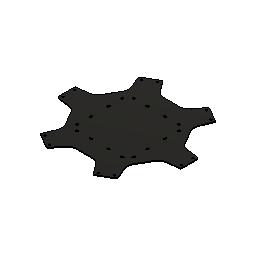
F550 Bottom Plate v5 (Autodesk Fusion 360 design; units mm, degrees)
Autodesk Fusion 360 part; units mm, degrees
sketch "Sketch1" plane through (0, 0, 0) normal (0, 0, 1) x (1, 0, 0)
  circle A0 centre (0, 0) radius 275 construction
  line L0 (-110, -15.85) -> (-110, 15.85)
  circle A1 centre (-105, 10.5) radius 1.75
  circle A2 centre (-105, -10.5) radius 1.75
  line L1 (-105, 10.5) -> (-105, -10.5) construction
  line L2 (0, 0) -> (-67.55, 39)
  line L3 (0, 0) -> (-67.55, -39)
  line L4 (0, 0) -> (-105, 0) construction
  line L5 (-110, -15.85) -> (-87.3994, -18.594)
  line L6 (-67.55, -39) -> (-74.3532, -27.2164)
  arc A3 (-74.3532, -27.2164) -> (-87.3994, -18.594) centre (-89.5087, -35.9664) ccw
  line L7 (-110, 15.85) -> (-87.3994, 18.594)
  arc A4 (-87.3994, 18.594) -> (-74.3532, 27.2164) centre (-89.5087, 35.9664) ccw
  line L8 (-67.55, 39) -> (-74.3532, 27.2164)
  point P0 (-110, 0)
  point P1 (-105, 0)
  point P2 (-275, 0)
  point P3 (-107, -10)
  point P4 (-107, 10)
  point P5 (-107, 0)
  dimension "d1" = 550
  dimension "d2" = 21
  dimension "d3" = 5
  dimension "d5" = 170
  dimension "d6" = 3.5
  dimension "d7" = 31.7
  dimension "d8" = 30
  dimension "d9" = 30
  dimension "d10" = 78
  dimension "d13" = 20
  dimension "d30" = 105
  dimension "d56" = 17.5
  constraint coincident A0.centre L2.start
  constraint vertical L0
  constraint midpoint L0 P0
  constraint horizontal A0.centre P0
  constraint vertical A1.centre A2.centre
  constraint coincident A1.centre L1.start
  constraint coincident A2.centre L1.end
  constraint midpoint L1 P1
  constraint coincident A0 P2
  constraint horizontal A0.centre P2
  constraint equal A1 A2
  constraint coincident P1 L4.end
  constraint horizontal A0.centre P1
  constraint equal L2 L3
  constraint perpendicular L3 L6
  constraint tangent L6 A3
  constraint tangent L5 A3
  constraint symmetric L0.start L4 L0.end
  constraint symmetric L3.end L4 L2.end
  constraint symmetric L4 L5.end L7.end
  constraint symmetric L4 L6.end A4.end
  constraint symmetric L4 A3 A4
  constraint coincident L4 P5
  measures "d1" diameter of A0
  measures "d2" distance of A1.centre A2.centre
  measures "d3" distance of L0 L1
  measures "d5" distance of L1 P2
  measures "d6" diameter of A1
  measures "d7" distance of L0.start L0.end
  measures "d8" angle of L3 L4
  measures "d9" angle of L2 L4
  measures "d10" distance of A0.centre L2.end
  measures "d13" distance of P3 P4
  measures "d30" distance of L1 A0.centre
  measures "d56" radius of A4
extrude "Extrude1" add sketch "Sketch1" along normal blind 1.5 makes body 1
fillet "Fillet1" radius 2 2 edges at (-110, 15.85, 0.75) (-110, -15.85, 0.75) on bodies 1
pattern_circular "C-Pattern1" count 6 over 360 about axis through (0, 0, 1.75) along (0, 0, 1) of bodies 1 makes body 2 at (-25.2134, -43.671, 0) makes body 3 at (25.2134, -43.671, 0) makes body 4 at (50.4269, 0, 0) makes body 5 at (25.2134, 43.671, 0) makes body 6 at (-25.2134, 43.671, 0)
combine "Combine1" operation add target body 1 tool bodies 2 3 4 5 6
sketch "Sketch3" plane through (0, 0, 1.5) normal (0, 0, 1) x (-1, 0, 0)
  circle A0 centre (61.5933, -85.6827) radius 1.75
  circle A1 centre (43.4067, -96.1827) radius 1.75
  circle A2 centre (-43.4067, -96.1827) radius 1.75
  circle A3 centre (-61.5933, -85.6827) radius 1.75
  circle A4 centre (-105, -10.5) radius 1.75
  circle A5 centre (-105, 10.5) radius 1.75
  circle A6 centre (-61.5933, 85.6827) radius 1.75
  circle A7 centre (-43.4067, 96.1827) radius 1.75
  circle A8 centre (43.4067, 96.1827) radius 1.75
  circle A9 centre (61.5933, 85.6827) radius 1.75
  arc A10 (110, 14.0781) -> (108.2411, 16.0636) centre (108, 14.0781) ccw
  line L0 (108.2411, 16.0636) -> (87.3994, 18.594)
  arc A11 (74.3532, 27.2164) -> (87.3994, 18.594) centre (89.5087, 35.9664) ccw
  line L1 (74.3532, 27.2164) -> (60.7467, 50.7836)
  arc A12 (59.8026, 66.3931) -> (60.7467, 50.7836) centre (75.9022, 59.5336) ccw
  line L2 (59.8026, 66.3931) -> (68.032, 85.7077)
  arc A13 (68.032, 85.7077) -> (67.192, 88.2237) centre (66.192, 86.4917) ccw
  line L3 (67.192, 88.2237) -> (42.808, 102.3019)
  arc A14 (42.808, 102.3019) -> (40.2091, 101.7713) centre (41.808, 100.5698) ccw
  line L4 (40.2091, 101.7713) -> (27.5968, 84.9871)
  arc A15 (13.6065, 78) -> (27.5968, 84.9871) centre (13.6065, 95.5) ccw
  line L5 (13.6065, 78) -> (-13.6065, 78)
  arc A16 (-27.5968, 84.9871) -> (-13.6065, 78) centre (-13.6065, 95.5) ccw
  line L6 (-27.5968, 84.9871) -> (-40.2091, 101.7713)
  arc A17 (-40.2091, 101.7713) -> (-42.808, 102.3019) centre (-41.808, 100.5698) ccw
  line L7 (-42.808, 102.3019) -> (-67.192, 88.2237)
  arc A18 (-67.192, 88.2237) -> (-68.032, 85.7077) centre (-66.192, 86.4917) ccw
  line L8 (-68.032, 85.7077) -> (-59.8026, 66.3931)
  arc A19 (-60.7467, 50.7836) -> (-59.8026, 66.3931) centre (-75.9022, 59.5336) ccw
  line L9 (-60.7467, 50.7836) -> (-74.3532, 27.2164)
  arc A20 (-87.3994, 18.594) -> (-74.3532, 27.2164) centre (-89.5087, 35.9664) ccw
  line L10 (-87.3994, 18.594) -> (-108.2411, 16.0636)
  arc A21 (-108.2411, 16.0636) -> (-110, 14.0781) centre (-108, 14.0781) ccw
  line L11 (-110, 14.0781) -> (-110, -14.0781)
  arc A22 (-110, -14.0781) -> (-108.2411, -16.0636) centre (-108, -14.0781) ccw
  line L12 (-108.2411, -16.0636) -> (-87.3994, -18.594)
  arc A23 (-74.3532, -27.2164) -> (-87.3994, -18.594) centre (-89.5087, -35.9664) ccw
  line L13 (-74.3532, -27.2164) -> (-60.7467, -50.7836)
  arc A24 (-59.8026, -66.3931) -> (-60.7467, -50.7836) centre (-75.9022, -59.5336) ccw
  line L14 (-59.8026, -66.3931) -> (-68.032, -85.7077)
  arc A25 (-68.032, -85.7077) -> (-67.192, -88.2237) centre (-66.192, -86.4917) ccw
  line L15 (-67.192, -88.2237) -> (-42.808, -102.3019)
  arc A26 (-42.808, -102.3019) -> (-40.2091, -101.7713) centre (-41.808, -100.5698) ccw
  line L16 (-40.2091, -101.7713) -> (-27.5968, -84.9871)
  arc A27 (-13.6065, -78) -> (-27.5968, -84.9871) centre (-13.6065, -95.5) ccw
  line L17 (-13.6065, -78) -> (13.6065, -78)
  arc A28 (27.5968, -84.9871) -> (13.6065, -78) centre (13.6065, -95.5) ccw
  line L18 (27.5968, -84.9871) -> (40.2091, -101.7713)
  arc A29 (40.2091, -101.7713) -> (42.808, -102.3019) centre (41.808, -100.5698) ccw
  line L19 (42.808, -102.3019) -> (67.192, -88.2237)
  arc A30 (67.192, -88.2237) -> (68.032, -85.7077) centre (66.192, -86.4917) ccw
  line L20 (68.032, -85.7077) -> (59.8026, -66.3931)
  arc A31 (60.7467, -50.7836) -> (59.8026, -66.3931) centre (75.9022, -59.5336) ccw
  line L21 (60.7467, -50.7836) -> (74.3532, -27.2164)
  arc A32 (87.3994, -18.594) -> (74.3532, -27.2164) centre (89.5087, -35.9664) ccw
  line L22 (87.3994, -18.594) -> (108.2411, -16.0636)
  arc A33 (108.2411, -16.0636) -> (110, -14.0781) centre (108, -14.0781) ccw
  line L23 (110, -14.0781) -> (110, 14.0781)
  circle A34 centre (105, -10.5) radius 1.75
  circle A35 centre (105, 10.5) radius 1.75
  line L24 (41.25, 51.75) -> (39.25, 51.75)
  arc A36 (39.25, 51.75) -> (39.25, 48.75) centre (39.25, 50.25) ccw
  line L25 (39.25, 48.75) -> (41.25, 48.75)
  arc A37 (41.25, 48.75) -> (41.25, 51.75) centre (41.25, 50.25) ccw
  line L26 (42.75, 50.25) -> (37.75, 50.25) construction
  line L27 (16.75, 51.75) -> (14.75, 51.75)
  arc A38 (14.75, 51.75) -> (14.75, 48.75) centre (14.75, 50.25) ccw
  line L28 (14.75, 48.75) -> (16.75, 48.75)
  arc A39 (16.75, 48.75) -> (16.75, 51.75) centre (16.75, 50.25) ccw
  line L29 (18.25, 50.25) -> (13.25, 50.25) construction
  line L30 (0, 78) -> (0, -78) construction
  line L31 (-18.25, 50.25) -> (-13.25, 50.25) construction
  line L32 (-42.75, 50.25) -> (-37.75, 50.25) construction
  arc A40 (-16.75, 51.75) -> (-16.75, 48.75) centre (-16.75, 50.25) ccw
  line L33 (-41.25, 51.75) -> (-39.25, 51.75)
  line L34 (-39.25, 48.75) -> (-41.25, 48.75)
  line L35 (-14.75, 48.75) -> (-16.75, 48.75)
  arc A41 (-14.75, 48.75) -> (-14.75, 51.75) centre (-14.75, 50.25) ccw
  arc A42 (-39.25, 48.75) -> (-39.25, 51.75) centre (-39.25, 50.25) ccw
  arc A43 (-41.25, 51.75) -> (-41.25, 48.75) centre (-41.25, 50.25) ccw
  line L36 (-16.75, 51.75) -> (-14.75, 51.75)
  line L37 (-50.25, -42.75) -> (-50.25, -37.75) construction
  line L38 (-50.25, 42.75) -> (-50.25, 37.75) construction
  line L39 (-51.75, -41.25) -> (-51.75, -39.25)
  arc A44 (-48.75, 41.25) -> (-51.75, 41.25) centre (-50.25, 41.25) ccw
  arc A45 (-51.75, -16.75) -> (-48.75, -16.75) centre (-50.25, -16.75) ccw
  line L40 (-50.25, -18.25) -> (-50.25, -13.25) construction
  line L41 (-50.25, 18.25) -> (-50.25, 13.25) construction
  arc A46 (-48.75, -39.25) -> (-51.75, -39.25) centre (-50.25, -39.25) ccw
  line L42 (-48.75, -39.25) -> (-48.75, -41.25)
  line L43 (-51.75, -16.75) -> (-51.75, -14.75)
  arc A47 (-51.75, -41.25) -> (-48.75, -41.25) centre (-50.25, -41.25) ccw
  line L44 (-48.75, 14.75) -> (-48.75, 16.75)
  arc A48 (-51.75, 14.75) -> (-48.75, 14.75) centre (-50.25, 14.75) ccw
  arc A49 (-48.75, -14.75) -> (-51.75, -14.75) centre (-50.25, -14.75) ccw
  line L45 (-48.75, 39.25) -> (-48.75, 41.25)
  arc A50 (-48.75, 16.75) -> (-51.75, 16.75) centre (-50.25, 16.75) ccw
  line L46 (-51.75, 41.25) -> (-51.75, 39.25)
  line L47 (-51.75, 16.75) -> (-51.75, 14.75)
  line L48 (-48.75, -14.75) -> (-48.75, -16.75)
  arc A51 (-51.75, 39.25) -> (-48.75, 39.25) centre (-50.25, 39.25) ccw
  line L49 (42.75, -50.25) -> (37.75, -50.25) construction
  line L50 (-42.75, -50.25) -> (-37.75, -50.25) construction
  line L51 (41.25, -51.75) -> (39.25, -51.75)
  arc A52 (-41.25, -48.75) -> (-41.25, -51.75) centre (-41.25, -50.25) ccw
  arc A53 (16.75, -51.75) -> (16.75, -48.75) centre (16.75, -50.25) ccw
  line L52 (18.25, -50.25) -> (13.25, -50.25) construction
  line L53 (-18.25, -50.25) -> (-13.25, -50.25) construction
  arc A54 (39.25, -48.75) -> (39.25, -51.75) centre (39.25, -50.25) ccw
  line L54 (39.25, -48.75) -> (41.25, -48.75)
  line L55 (16.75, -51.75) -> (14.75, -51.75)
  arc A55 (41.25, -51.75) -> (41.25, -48.75) centre (41.25, -50.25) ccw
  line L56 (-14.75, -48.75) -> (-16.75, -48.75)
  arc A56 (-14.75, -51.75) -> (-14.75, -48.75) centre (-14.75, -50.25) ccw
  arc A57 (14.75, -48.75) -> (14.75, -51.75) centre (14.75, -50.25) ccw
  line L57 (-39.25, -48.75) -> (-41.25, -48.75)
  arc A58 (-16.75, -48.75) -> (-16.75, -51.75) centre (-16.75, -50.25) ccw
  line L58 (-41.25, -51.75) -> (-39.25, -51.75)
  line L59 (-16.75, -51.75) -> (-14.75, -51.75)
  line L60 (14.75, -48.75) -> (16.75, -48.75)
  arc A59 (-39.25, -51.75) -> (-39.25, -48.75) centre (-39.25, -50.25) ccw
  line L61 (50.25, 42.75) -> (50.25, 37.75) construction
  line L62 (50.25, -42.75) -> (50.25, -37.75) construction
  line L63 (51.75, 41.25) -> (51.75, 39.25)
  arc A60 (48.75, -41.25) -> (51.75, -41.25) centre (50.25, -41.25) ccw
  arc A61 (51.75, 16.75) -> (48.75, 16.75) centre (50.25, 16.75) ccw
  line L64 (50.25, 18.25) -> (50.25, 13.25) construction
  line L65 (50.25, -18.25) -> (50.25, -13.25) construction
  arc A62 (48.75, 39.25) -> (51.75, 39.25) centre (50.25, 39.25) ccw
  line L66 (48.75, 39.25) -> (48.75, 41.25)
  line L67 (51.75, 16.75) -> (51.75, 14.75)
  arc A63 (51.75, 41.25) -> (48.75, 41.25) centre (50.25, 41.25) ccw
  line L68 (48.75, -14.75) -> (48.75, -16.75)
  arc A64 (51.75, -14.75) -> (48.75, -14.75) centre (50.25, -14.75) ccw
  arc A65 (48.75, 14.75) -> (51.75, 14.75) centre (50.25, 14.75) ccw
  line L69 (48.75, -39.25) -> (48.75, -41.25)
  arc A66 (48.75, -16.75) -> (51.75, -16.75) centre (50.25, -16.75) ccw
  line L70 (51.75, -41.25) -> (51.75, -39.25)
  line L71 (51.75, -16.75) -> (51.75, -14.75)
  line L72 (48.75, 14.75) -> (48.75, 16.75)
  arc A67 (51.75, -39.25) -> (48.75, -39.25) centre (50.25, -39.25) ccw
  dimension "d44" = 5
  dimension "d45" = 3
  dimension "d47" = 5
  dimension "d48" = 3
  dimension "d49" = 14.75
  dimension "d50" = 19.5
  dimension "d52" = 48.75
  dimension "d54" = 360
  constraint tangent L24 A36
  constraint tangent A36 L25
  constraint parallel L24 L25
  constraint tangent L25 A37
  constraint tangent L24 A37
  constraint midpoint A37 L26.start
  constraint midpoint A36 L26.end
  constraint horizontal L26
  constraint tangent L27 A38
  constraint tangent A38 L28
  constraint parallel L27 L28
  constraint tangent L28 A39
  constraint tangent L27 A39
  constraint midpoint A39 L29.start
  constraint midpoint A38 L29.end
  constraint horizontal L29
  constraint midpoint L5 L30.start
  constraint midpoint L17 L30.end
  constraint horizontal A36.centre A39.centre
  constraint symmetric L24.start L30 L33.start
  constraint symmetric L24.end L30 L33.end
  constraint symmetric A36.end L30 L34.start
  constraint symmetric L25.end L30 L34.end
  constraint symmetric A36 L30 A42
  constraint symmetric A37 L30 A43
  constraint symmetric L26.start L30 L32.start
  constraint symmetric L26.end L30 L32.end
  constraint symmetric L27.start L30 A40.start
  constraint symmetric L27.end L30 A41.end
  constraint symmetric A38.end L30 L35.start
  constraint symmetric L28.end L30 A40.end
  constraint symmetric A38 L30 A41
  constraint symmetric A39 L30 A40
  constraint symmetric L29.start L30 L31.start
  constraint symmetric L29.end L30 L31.end
  measures "d44" distance of L29.start L29.end
  measures "d45" distance of L27 L28
  measures "d47" distance of L26.start L26.end
  measures "d48" distance of L24 L25
  measures "d49" distance of A38.centre L30
  measures "d50" horizontal distance of L26.end L29.start
  measures "d52" distance of origin L28
extrude "Extrude3" cut sketch "Sketch3" against normal through all contours L24 A36 L25 A37 | L27 A38 L28 A39 | A40 L35 A41 L36 | L33 L34 A42 A43 | L39 A46 L42 A47 | A44 L45 L46 A51 | A45 L43 A49 L48 | L44 A48 A50 L47 | L51 A54 L54 A55 | A52 L57 L58 A59 | A53 L55 A57 L60 | L56 A56 A58 L59 | L63 A62 L66 A63 | A60 L69 L70 A67 | A61 L67 A65 L72 | L68 A64 A66 L71 bodies 1
equation "d9 = d8"
equation "d10 = ( 156 / 2 ) * 1 mm"
equation "d47 = d44"
equation "d48 = d45"
equation "d49 = ( 29.5 / 2 ) * 1 mm"
equation "d52 = ( 97.5 / 2 ) * 1 mm"
